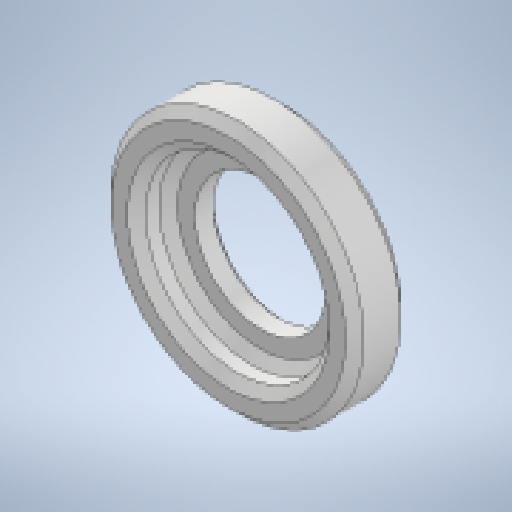
# Autodesk Inventor part: 托带轮
Saved by Autodesk Inventor 2025.1 (Build 291241000, 241)
## iProperties
Created: 2025-08-31
Part Number: 托带轮
Material: 常规
Document SubType Name: Modeling
Designer: Piw
Density: 1 g/cm^3
Appearance: 默认
Author: Piw
Autodesk Inventor part; units mm, degrees
ref_plane "YZ Plane" through (0, 0, 0) normal (1, 0, 0) x (0, 1, 0)
sketch "草图1" plane through (0, 0, 0) normal (0, 0, 1) x (1, 0, 0)
  circle A0 centre (0, 63.5912) radius 4 projected
  circle A1 centre (0, 63.5912) radius 14.25
  circle A2 centre (0, 63.5912) radius 27.5
  point P0 (0, 0)
  dimension "d0" = 28.5
  dimension "d1" = 55
  constraints: 2 centre point, 2 coincident
  measures "d0" diameter of A1
  measures "d1" diameter of A2
ref_plane "工作平面1" through (-67.7438, -99.1526, 12) normal (0, 0, 1) x (0.7634103, -0.6459139, 0)
extrude "拉伸1" add sketch "草图1" along normal up to surface (12 mm away) contours A2
chamfer "倒角1" distance 2 angle 45 2 edges at (-27.5, 63.5912, 12) (-27.5, 63.5912, 0)
sketch "草图2" plane through (0, 63.5912, 12) normal (0, 0, 1) x (1, 0, 0)
  circle A0 centre (0, 0) radius 14.25 projected
  circle A1 centre (0, 0) radius 20
  point P0 (0, -63.5912)
  dimension "d7" = 40
  constraints: 1 centre point, 1 coincident
  measures "d7" diameter of A1
ref_plane "工作平面2" through (-24.6728, 38.9185, 5) normal (0, 0, 1) x (1, 0, 0)
extrude "拉伸2" cut sketch "草图2" against normal up to surface (7 mm away)
chamfer "倒角2" distance 2 angle 45 2 edges at (-20, 63.5912, 5) (-20, 63.5912, 12)
chamfer "倒角3" distance 1 angle 45 1 edges at (-14.25, 63.5912, 0)
